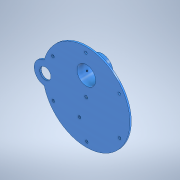
# Autodesk Inventor part: filterTop
Saved by Autodesk Inventor 2022.2 (Build 262287000, 287)
## iProperties
Created: 2020-04-12
Part Number: filterTop
Material: PBT Plastic
Document SubType Name: Modeling
Designer: robst
Density: 1.31 g/cm^3
Appearance: Cyan
Author: robst
Autodesk Inventor part; units mm, degrees
ref_plane "YZ Plane" through (0, 0, 0) normal (1, 0, 0) x (0, 1, 0)
ref_plane "XY Plane" through (0, 0, 0) normal (0, 0, 1) x (1, 0, 0)
sketch "Sketch7" plane through (0, 0, 0) normal (0, 0, 1) x (1, 0, 0)
  circle A0 centre (0, 0) radius 76.2
  dimension "d15" = 152.4
  constraints: 1 centre point, 1 coincident
  measures "d15" diameter of A0
extrude "Extrusion4" add sketch "Sketch7" against normal blind 2.54
sketch "Sketch8" plane through (0, 0, 0) normal (0, 0, 1) x (1, 0, 0)
  circle A0 centre (0, 33.1656) radius 16.383
  point P0 (0, 0)
  dimension "d18" = 33.1656
  dimension "d19" = 32.766
  constraints: 1 centre point
  measures "d18" distance of A0.centre point (0, 0)
  measures "d19" diameter of A0
extrude "Extrusion5" cut sketch "Sketch8" against normal through all
sketch "Sketch9" plane through (0, 0, -2.54) normal (0, 0, -1) x (-1, 0, 0)
  arc A0 (-49.5486, 0) -> (49.5486, 0) centre (0, 0) ccw construction
  circle A1 centre (0, 33.1656) radius 16.383 construction
  line L0 (49.5486, 0) -> (-49.5486, 0) construction
  line L1 (46.2132, 5.178) -> (51.5596, 5.7294)
  line L2 (51.5596, 5.7294) -> (51.3498, 7.7638)
  line L3 (51.3498, 7.7638) -> (52.0673, 7.8378)
  line L4 (52.0673, 7.8378) -> (52.57, 2.9631)
  line L5 (52.57, 2.9631) -> (51.8525, 2.8891)
  line L6 (51.8525, 2.8891) -> (51.6427, 4.9235)
  line L7 (51.6427, 4.9235) -> (46.2963, 4.3721)
  line L8 (46.2963, 4.3721) -> (46.2132, 5.178)
  spline S0 degree 2 poles (51.8686, -2.6687) (51.4588, -3.009) (50.2681, -3.3782) (49.5074, -3.3678) knots 0 0 0 1 2 2 2
  spline S1 degree 2 poles (49.5074, -3.3678) (48.7665, -3.3577) (47.5713, -2.966) (47.171, -2.6049) knots 0 0 0 1 2 2 2
  spline S2 degree 2 poles (47.171, -2.6049) (46.7513, -2.2237) (46.3598, -1.2253) (46.3679, -0.6276) knots 0 0 0 1 2 2 2
  spline S3 degree 2 poles (46.3679, -0.6276) (46.3763, -0.0102) (46.8096, 0.972) (47.2245, 1.327) knots 0 0 0 1 2 2 2
  spline S4 degree 2 poles (47.2245, 1.327) (47.6343, 1.6722) (48.8298, 2.0315) (49.5806, 2.0213) knots 0 0 0 1 2 2 2
  spline S5 degree 2 poles (49.5806, 2.0213) (50.3463, 2.0109) (51.5069, 1.6147) (51.922, 1.2582) knots 0 0 0 1 2 2 2
  spline S6 degree 2 poles (51.922, 1.2582) (52.3222, 0.8971) (52.7285, -0.1015) (52.7202, -0.714) knots 0 0 0 1 2 2 2
  spline S7 degree 2 poles (52.7202, -0.714) (52.7118, -1.3364) (52.2635, -2.3282) (51.8686, -2.6687) knots 0 0 0 1 2 2 2
  spline S8 degree 2 poles (49.5189, -2.5232) (50.1215, -2.5313) (51.0587, -2.2822) (51.3681, -2.0493) knots 0 0 0 1 2 2 2
  spline S9 degree 2 poles (51.3681, -2.0493) (51.6876, -1.8115) (52.013, -1.1342) (52.0187, -0.7094) knots 0 0 0 1 2 2 2
  spline S10 degree 2 poles (52.0187, -0.7094) (52.0247, -0.2698) (51.7274, 0.3963) (51.4049, 0.6527) knots 0 0 0 1 2 2 2
  spline S11 degree 2 poles (51.4049, 0.6527) (51.0969, 0.8989) (50.1619, 1.1685) (49.5692, 1.1766) knots 0 0 0 1 2 2 2
  spline S12 degree 2 poles (49.5692, 1.1766) (48.3689, 1.1929) (47.0807, 0.2025) (47.0693, -0.6421) knots 0 0 0 1 2 2 2
  spline S13 degree 2 poles (47.0693, -0.6421) (47.0578, -1.4868) (48.3186, -2.5068) (49.5189, -2.5232) knots 0 0 0 1 2 2 2
  spline S14 degree 2 poles (50.0769, -8.5692) (49.6849, -8.5192) (49.0149, -8.1498) (48.8018, -7.8686) knots 0 0 0 1 2 2 2
  spline S15 degree 2 poles (48.8018, -7.8686) (48.5331, -7.5155) (48.3228, -6.6271) (48.4054, -5.9803) knots 0 0 0 1 2 2 2
  line L9 (48.4054, -5.9803) -> (48.4924, -5.2992)
  line L10 (48.4924, -5.2992) -> (46.2382, -5.0114)
  line L11 (46.2382, -5.0114) -> (46.3408, -4.2077)
  line L12 (46.3408, -4.2077) -> (52.3878, -4.9797)
  line L13 (52.3878, -4.9797) -> (52.1938, -6.4988)
  spline S16 degree 2 poles (52.1938, -6.4988) (52.125, -7.0378) (51.8523, -7.7699) (51.6144, -8.0334) knots 0 0 0 1 2 2 2
  spline S17 degree 2 poles (51.6144, -8.0334) (51.341, -8.3421) (50.5816, -8.6336) (50.0769, -8.5692) knots 0 0 0 1 2 2 2
  spline S18 degree 2 poles (50.1594, -7.7281) (50.473, -7.7682) (50.9611, -7.6114) (51.1363, -7.4096) knots 0 0 0 1 2 2 2
  spline S19 degree 2 poles (51.1363, -7.4096) (51.2881, -7.2348) (51.4561, -6.7383) (51.5042, -6.361) knots 0 0 0 1 2 2 2
  line L14 (51.5042, -6.361) -> (51.5893, -5.6945)
  line L15 (51.5893, -5.6945) -> (49.1784, -5.3867)
  line L16 (49.1784, -5.3867) -> (49.1083, -5.9356)
  spline S20 degree 2 poles (49.1083, -5.9356) (49.0458, -6.4256) (49.1256, -7.0483) (49.3064, -7.2706) knots 0 0 0 1 2 2 2
  spline S21 degree 2 poles (49.3064, -7.2706) (49.4646, -7.4751) (49.8703, -7.6912) (50.1594, -7.7281) knots 0 0 0 1 2 2 2
  line L17 (49.7294, -17.3105) -> (44.4787, -13.5689)
  line L18 (44.4787, -13.5689) -> (44.7266, -12.7304)
  line L19 (44.7266, -12.7304) -> (51.1677, -12.4453)
  line L20 (51.1677, -12.4453) -> (50.9212, -13.279)
  line L21 (50.9212, -13.279) -> (45.5864, -13.4637)
  line L22 (45.5864, -13.4637) -> (49.9632, -16.5194)
  line L23 (49.9632, -16.5194) -> (49.7294, -17.3105)
  spline S22 degree 2 poles (45.0636, -20.6915) (43.5474, -20.0663) (42.4905, -18.5993) (42.869, -17.6813) knots 0 0 0 1 2 2 2
  spline S23 degree 2 poles (42.869, -17.6813) (43.2531, -16.7496) (45.0606, -16.4743) (46.5448, -17.0863) knots 0 0 0 1 2 2 2
  spline S24 degree 2 poles (46.5448, -17.0863) (48.0702, -17.7152) (49.118, -19.1785) (48.7376, -20.1011) knots 0 0 0 1 2 2 2
  spline S25 degree 2 poles (48.7376, -20.1011) (48.3554, -21.0282) (46.5342, -21.2979) (45.0636, -20.6915) knots 0 0 0 1 2 2 2
  spline S26 degree 2 poles (43.7457, -19.0153) (43.9791, -19.2398) (44.8, -19.6851) (45.38, -19.9243) knots 0 0 0 1 2 2 2
  spline S27 degree 2 poles (45.38, -19.9243) (45.96, -20.1634) (46.8517, -20.4242) (47.1865, -20.4287) knots 0 0 0 1 2 2 2
  spline S28 degree 2 poles (47.1865, -20.4287) (47.5213, -20.4332) (47.982, -20.1582) (48.1119, -19.8431) knots 0 0 0 1 2 2 2
  spline S29 degree 2 poles (48.1119, -19.8431) (48.2419, -19.528) (48.1126, -18.9991) (47.8647, -18.758) knots 0 0 0 1 2 2 2
  spline S30 degree 2 poles (47.8647, -18.758) (47.6241, -18.5251) (46.7811, -18.0814) (46.2285, -17.8535) knots 0 0 0 1 2 2 2
  spline S31 degree 2 poles (46.2285, -17.8535) (45.6348, -17.6087) (44.81, -17.3541) (44.4505, -17.3448) knots 0 0 0 1 2 2 2
  spline S32 degree 2 poles (44.4505, -17.3448) (44.113, -17.3339) (43.6302, -17.6104) (43.4947, -17.9393) knots 0 0 0 1 2 2 2
  spline S33 degree 2 poles (43.4947, -17.9393) (43.3666, -18.2498) (43.4959, -18.7787) (43.7457, -19.0153) knots 0 0 0 1 2 2 2
  line L24 (40.2855, -23.2804) -> (41.6835, -20.6556)
  line L25 (41.6835, -20.6556) -> (42.2329, -20.9482)
  line L26 (42.2329, -20.9482) -> (41.7127, -21.9249)
  line L27 (41.7127, -21.9249) -> (45.3186, -23.8453)
  line L28 (45.3186, -23.8453) -> (45.8387, -22.8686)
  line L29 (45.8387, -22.8686) -> (46.3314, -23.1311)
  spline S34 degree 2 poles (46.3314, -23.1311) (46.0365, -23.6848) (46.0718, -24.3752) (46.4892, -24.6423) knots 0 0 0 1 2 2 2
  line L30 (46.4892, -24.6423) -> (46.192, -25.2004)
  line L31 (46.192, -25.2004) -> (41.3435, -22.6181)
  line L32 (41.3435, -22.6181) -> (40.8349, -23.573)
  line L33 (40.8349, -23.573) -> (40.2855, -23.2804)
  spline S35 degree 2 poles (39.2798, -32.2215) (38.9639, -31.9841) (38.5644, -31.3316) (38.5183, -30.9818) knots 0 0 0 1 2 2 2
  spline S36 degree 2 poles (38.5183, -30.9818) (38.4595, -30.5421) (38.7162, -29.6659) (39.108, -29.1447) knots 0 0 0 1 2 2 2
  line L34 (39.108, -29.1447) -> (39.5205, -28.5957)
  line L35 (39.5205, -28.5957) -> (37.704, -27.2305)
  line L36 (37.704, -27.2305) -> (38.1907, -26.5828)
  line L37 (38.1907, -26.5828) -> (43.0639, -30.2453)
  line L38 (43.0639, -30.2453) -> (42.1438, -31.4695)
  spline S37 degree 2 poles (42.1438, -31.4695) (41.8173, -31.9039) (41.2181, -32.4052) (40.8811, -32.5165) knots 0 0 0 1 2 2 2
  spline S38 degree 2 poles (40.8811, -32.5165) (40.4907, -32.6495) (39.6866, -32.5272) (39.2798, -32.2215) knots 0 0 0 1 2 2 2
  spline S39 degree 2 poles (39.7676, -31.5314) (40.0203, -31.7213) (40.5221, -31.8265) (40.7742, -31.7379) knots 0 0 0 1 2 2 2
  spline S40 degree 2 poles (40.7742, -31.7379) (40.9926, -31.661) (41.3842, -31.3126) (41.6127, -31.0086) knots 0 0 0 1 2 2 2
  line L39 (41.6127, -31.0086) -> (42.0164, -30.4715)
  line L40 (42.0164, -30.4715) -> (40.0734, -29.0113)
  line L41 (40.0734, -29.0113) -> (39.741, -29.4536)
  spline S41 degree 2 poles (39.741, -29.4536) (39.4442, -29.8485) (39.2055, -30.4292) (39.2527, -30.7118) knots 0 0 0 1 2 2 2
  spline S42 degree 2 poles (39.2527, -30.7118) (39.289, -30.9677) (39.5346, -31.3563) (39.7676, -31.5314) knots 0 0 0 1 2 2 2
  line L42 (36.8288, -37.6338) -> (33.792, -31.9464)
  line L43 (33.792, -31.9464) -> (34.3872, -31.3058)
  line L44 (34.3872, -31.3058) -> (40.2821, -33.917)
  line L45 (40.2821, -33.917) -> (39.6903, -34.554)
  line L46 (39.6903, -34.554) -> (34.8308, -32.3451)
  line L47 (34.8308, -32.3451) -> (37.3904, -37.0294)
  line L48 (37.3904, -37.0294) -> (36.8288, -37.6338)
  spline S43 degree 2 poles (31.1459, -38.585) (30.0663, -37.3503) (29.7728, -35.5662) (30.5203, -34.9126) knots 0 0 0 1 2 2 2
  spline S44 degree 2 poles (30.5203, -34.9126) (31.279, -34.2492) (33.0201, -34.807) (34.0769, -36.0157) knots 0 0 0 1 2 2 2
  spline S45 degree 2 poles (34.0769, -36.0157) (35.163, -37.2578) (35.45, -39.0345) (34.6988, -39.6914) knots 0 0 0 1 2 2 2
  spline S46 degree 2 poles (34.6988, -39.6914) (33.9438, -40.3515) (32.193, -39.7825) (31.1459, -38.585) knots 0 0 0 1 2 2 2
  spline S47 degree 2 poles (30.7117, -36.4973) (30.8208, -36.8022) (31.3577, -37.5664) (31.7707, -38.0387) knots 0 0 0 1 2 2 2
  spline S48 degree 2 poles (31.7707, -38.0387) (32.1837, -38.511) (32.8661, -39.1414) (33.1639, -39.2944) knots 0 0 0 1 2 2 2
  spline S49 degree 2 poles (33.1639, -39.2944) (33.4618, -39.4474) (33.9967, -39.4062) (34.2533, -39.1819) knots 0 0 0 1 2 2 2
  spline S50 degree 2 poles (34.2533, -39.1819) (34.5099, -38.9575) (34.6295, -38.4264) (34.5148, -38.1001) knots 0 0 0 1 2 2 2
  spline S51 degree 2 poles (34.5148, -38.1001) (34.403, -37.7845) (33.8456, -37.012) (33.4521, -36.562) knots 0 0 0 1 2 2 2
  spline S52 degree 2 poles (33.4521, -36.562) (33.0294, -36.0785) (32.4041, -35.4835) (32.0863, -35.3151) knots 0 0 0 1 2 2 2
  spline S53 degree 2 poles (32.0863, -35.3151) (31.7889, -35.1552) (31.2336, -35.188) (30.9658, -35.4221) knots 0 0 0 1 2 2 2
  spline S54 degree 2 poles (30.9658, -35.4221) (30.7129, -35.6432) (30.5933, -36.1743) (30.7117, -36.4973) knots 0 0 0 1 2 2 2
  line L49 (25.4656, -38.9549) -> (28.5249, -36.77)
  line L50 (28.5249, -36.77) -> (29.0274, -37.4735)
  spline S55 degree 2 poles (29.0274, -37.4735) (28.9188, -38.0185) (28.7424, -39.0125) (28.6821, -39.523) knots 0 0 0 1 2 2 2
  spline S56 degree 2 poles (28.6821, -39.523) (28.5603, -40.5509) (28.6802, -41.5944) (28.9645, -41.9924) knots 0 0 0 1 2 2 2
  spline S57 degree 2 poles (28.9645, -41.9924) (29.1138, -42.2014) (29.4663, -42.4231) (29.6547, -42.4404) knots 0 0 0 1 2 2 2
  spline S58 degree 2 poles (29.6547, -42.4404) (29.8431, -42.4576) (30.2204, -42.3399) (30.4053, -42.2078) knots 0 0 0 1 2 2 2
  spline S59 degree 2 poles (30.4053, -42.2078) (30.5822, -42.0815) (30.8808, -41.7347) (30.9968, -41.5486) knots 0 0 0 1 2 2 2
  spline S60 degree 2 poles (30.9968, -41.5486) (31.0973, -41.3918) (31.2438, -41.0444) (31.284, -40.9307) knots 0 0 0 1 2 2 2
  line L51 (31.284, -40.9307) -> (31.3202, -40.9049)
  line L52 (31.3202, -40.9049) -> (31.8255, -41.6124)
  spline S61 degree 2 poles (31.8255, -41.6124) (31.6922, -41.8593) (31.0972, -42.5817) (30.7676, -42.8172) knots 0 0 0 1 2 2 2
  spline S62 degree 2 poles (30.7676, -42.8172) (30.0721, -43.3138) (28.7628, -43.138) (28.3149, -42.5109) knots 0 0 0 1 2 2 2
  spline S63 degree 2 poles (28.3149, -42.5109) (28.1053, -42.2174) (27.8918, -41.6294) (27.8631, -41.3342) knots 0 0 0 1 2 2 2
  spline S64 degree 2 poles (27.8631, -41.3342) (27.8286, -41.031) (27.874, -40.3551) (27.9206, -40.0122) knots 0 0 0 1 2 2 2
  spline S65 degree 2 poles (27.9206, -40.0122) (27.9901, -39.4466) (28.2354, -38.1666) (28.3124, -37.7899) knots 0 0 0 1 2 2 2
  line L53 (28.3124, -37.7899) -> (25.8762, -39.5297)
  line L54 (25.8762, -39.5297) -> (25.4656, -38.9549)
  constraints: 2 end point, 2 point on circle, 1 centre point, 1 coincident, 1 horizontal, 1 tangent, 1 other
extrude "DescriptionText" cut sketch "Sketch9" against normal blind 0.635
sketch "Sketch10" plane through (0, 0, -2.54) normal (0, 0, -1) x (-1, 0, 0)
  circle A0 centre (0, 33.1656) radius 16.383 projected
  circle A1 centre (0, 33.1656) radius 16.383
  circle A2 centre (0, 33.1656) radius 18.923
  point P0 (0, 0)
  dimension "d24" = 2.54
  constraints: 2 centre point, 2 coincident, 1 concentric
  measures "d24" radial gap between concentric circles of A0 A2
extrude "Extrusion7" add sketch "Sketch10" along normal blind 25.4
sketch "Sketch11" plane through (0, 0, -2.54) normal (0, 0, -1) x (-1, 0, 0)
  point P0 (0, 0)
  point P1 (0, 0)
  constraints: 1 coincident
hole "Hole1" at (0, 0, -2.54) direction (0, 0, 1) diameter 5.1054 end through all clearance for "Flat Head Machine Screw (82)" size "#10" standard "Ansi Unified Screw Threads"
sketch "Sketch12" plane through (0, 0, -2.54) normal (0, 0, -1) x (-1, 0, 0)
  circle A0 centre (0, 0) radius 2.5527 construction
  line L0 (0, 0) -> (76.2, 0) construction
  circle A1 centre (0, 0) radius 76.2 construction
  circle A2 centre (0, 0) radius 76.2 construction
  circle A3 centre (71.755, 0) radius 3.175
  dimension "d34" = 6.35
  dimension "d35" = 71.755
  constraints: 2 end point, 2 horizontal alignment, 1 centre point, 1 horizontal, 1 point on line, 1 other
  measures "d34" diameter of A3
  measures "d35" distance of A3.centre point (0, 0)
extrude "Extrusion8" cut sketch "Sketch12" against normal through all
sketch "Sketch13" plane through (0, 0, -2.54) normal (0, 0, -1) x (-1, 0, 0)
  circle A0 centre (0, 0) radius 76.2 projected
  circle A1 centre (71.755, 0) radius 3.175 projected
  arc A2 (74.3072, -16.8785) -> (74.3072, 16.8785) centre (71.755, 0) ccw
  arc A3 (73.658, -19.5178) -> (73.658, 19.5178) centre (71.755, 0) ccw
  circle A4 centre (0, 0) radius 2.5527 projected
  arc A5 (73.658, -19.5178) -> (73.658, 19.5178) centre (0, 0) ccw
  point P0 (76.0567, 4.671)
  point P1 (76.0567, -4.671)
  dimension "d38" = 17.0703
  dimension "d39" = 2.54
  constraints: 10 point on circle, 3 centre point, 3 coincident, 1 concentric, 1 other
  measures "d38" radius of A2
  measures "d39" radial gap between concentric circles of A3 A2
extrude "Extrusion9" add sketch "Sketch13" against normal up to surface (2.54 mm away) contours A0 A2 | A0 A3 A2 | A1
sketch "Sketch14" plane through (0, 0, 0) normal (0, 0, 1) x (1, 0, 0)
  circle A0 centre (0, 0) radius 2.5527 construction
  circle A1 centre (0, 0) radius 38.1 construction
  line L0 (0, 0) -> (0, -38.1) construction
  line L1 (0, 0) -> (-11.7735, -36.2353) construction
  dimension "d42" = 76.2
  dimension "d43" = 18
  constraints: 4 end point, 2 coincident, 2 point on circle, 1 centre point, 1 vertical
  measures "d42" diameter of A1
  measures "d43" angle of L1 L0
hole "Hole2" at (-11.7735, -36.2353, 0) direction (0, 0, -1) diameter 4.4958 end through all clearance for "Flat Head Machine Screw (82)" size "#8" standard "Ansi Unified Screw Threads"
sketch "Sketch15" plane through (0, 0, -2.54) normal (0, 0, -1) x (-1, 0, 0)
  circle A0 centre (0, 0) radius 2.5527 construction
  circle A1 centre (0, 0) radius 67.0077 construction
  line L0 (0, 0) -> (0, 67.0077) construction
  line L1 (0, 0.9037) -> (-57.6351, 34.1794) construction
  point P0 (-58.4178, -32.8238)
  point P1 (-0.7826, -67.0032)
  point P2 (57.6351, -34.1794)
  point P3 (58.4178, 32.8238)
  point P4 (0.7826, 67.0032)
  dimension "d51" = 134.0155
  dimension "d52" = 60
  dimension "d55" = 360
  constraints: 4 end point, 2 coincident, 2 point on circle, 1 centre point, 1 point on line, 1 vertical, 7 other
  measures "d51" diameter of A1
  measures "d52" angle of L1 L0
hole "MountingHoleSize8" at (57.6351, 34.1794, -2.54) at (58.4178, -32.8238, -2.54) at (0.7826, -67.0032, -2.54) at (-0.7826, 67.0032, -2.54) at (-58.4178, 32.8238, -2.54) at (-57.6351, -34.1794, -2.54) direction (0, 0, 1) diameter 4.4958 end through all clearance for "Flat Head Machine Screw (82)" size "#8" standard "Ansi Unified Screw Threads"
sketch "Sketch16" plane through (0, 0, -2.54) normal (0, 0, -1) x (-1, 0, 0)
  point P0 (0, 0)
  point P1 (71.755, 0)
  dimension "d64" = 71.755
  measures "d64" distance of point (71.755, 0) point (0, 0)
hole "Hole4" at (-71.755, 0, -2.54) direction (0, 0, 1) diameter 19.558 end through all
ref_plane "Work Plane1" through (0, 52.0886, -2.54) normal (0, 1, 0) x (-1, 0, 0)
sketch "Sketch17" plane through (0, 52.0886, -2.54) normal (0, 1, 0) x (-1, 0, 0)
  line L0 (-18.923, -25.4) -> (18.923, -25.4) projected
  line L1 (-76.2, 0) -> (73.658, 0) projected
  line L2 (18.923, 0) -> (18.923, -25.4) projected
  line L3 (-18.923, 0) -> (-18.923, -25.4) projected
  line L4 (0, -25.4) -> (0, 0) construction
  point P0 (0, 2.54)
  point P1 (0, -12.7)
  constraints: 2 end point, 2 midpoint, 1 point on line, 1 vertical
hole "ThreadHoleInEyepieceInsert" at (0, 52.0886, -15.24) direction (0, -1, 0) diameter 2.6416 end up to face face through (0, 33.1656, 0) facing (0, 0, -1) round with radius 16.383 far side no thread size "6-32 UNC" class "2B" standard "ANSI Unified Screw Threads"
pattern_circular "Circular PatternForEyepieceScrew" count 3 over 360 about axis through (0, 33.1656, 0) along (0, 0, -1) of "ThreadHoleInEyepieceInsert"
equation "\"d15\" = outsideDiameter"
equation "\"d16\" = wallThicknessForEyepieceHolder"
equation "\"d18\" = radiusForEyepieceHole"
equation "\"d19\" = eyepieceHoleInsideDiamter"
equation "\"height\" = 31.75"
equation "\"outerDiameter\" = 129.54"
equation "\"outerRadius\" = 0.5 * outerDiameter"
equation "\"centerHoleDiameter\" = 9.525"
equation "\"eyepieceHoleInsideDiamter\" = 32.766"
equation "\"radiusForEyepieceHole\" = 33.16561"
equation "\"wallThickness\" = 2.54"
equation "\"wallThicknessForEyepieceHolder\" = 2.54"
equation "\"outsideDiameter\" = 152.4"
body "Solid2"
body "Solid3"
